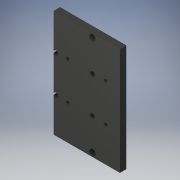
# Autodesk Inventor part: lidarCamMountv2
Saved by Autodesk Inventor 2017 (Build 210142000, 142)
## iProperties
Created: 2017-03-03
Part Number: lidarCamMountv2
Material: ABS Plastic
Document SubType Name: Modeling
Designer: Naga
Density: 1.06 g/cm^3
Appearance: Smooth - Black
Author: Naga
Autodesk Inventor part; units mm, degrees
ref_plane "YZ Plane" through (0, 0, 0) normal (1, 0, 0) x (0, 1, 0)
ref_plane "XZ Plane" through (0, 0, 0) normal (0, 1, 0) x (-1, 0, 0)
ref_plane "XY Plane" through (0, 0, 0) normal (0, 0, 1) x (1, 0, 0)
sketch "Sketch1" plane through (0, 0, 0) normal (0, 0, 1) x (1, 0, 0)
  line L0 (-33.3375, -53.975) -> (33.3375, -53.975)
  line L1 (33.3375, -53.975) -> (33.3375, 53.975)
  line L2 (33.3375, 53.975) -> (-33.3375, 53.975)
  line L3 (-33.3375, 53.975) -> (-33.3375, -53.975)
  line L4 (-33.3375, -53.975) -> (33.3375, 53.975) construction
  line L5 (33.3375, -53.975) -> (-33.3375, 53.975) construction
  point P0 (0, 0)
  dimension "d0" = 66.675
  dimension "d1" = 107.95
  constraints: 12 end point, 2 midpoint, 2 parallel, 1 horizontal, 1 perpendicular
  measures "d0" distance of L2.end L1.end
  measures "d1" distance of L1.end L0.end
extrude "Extrusion1" add sketch "Sketch1" along normal blind 6.35
sketch "Sketch3" plane through (0, 0, 6.35) normal (0, 0, 1) x (1, 0, 0)
  line L0 (-19.05, -19.05) -> (19.05, -19.05)
  line L1 (19.05, -19.05) -> (19.05, 19.05)
  line L2 (19.05, 19.05) -> (-19.05, 19.05)
  line L3 (-19.05, 19.05) -> (-19.05, -19.05)
  line L4 (-19.05, -19.05) -> (19.05, 19.05) construction
  line L5 (19.05, -19.05) -> (-19.05, 19.05) construction
  line L6 (0, 0) -> (-12.7, 0)
  line L7 (-31.115, -18.415) -> (5.715, -18.415)
  line L8 (5.715, -18.415) -> (5.715, 18.415)
  line L9 (5.715, 18.415) -> (-31.115, 18.415)
  line L10 (-31.115, 18.415) -> (-31.115, -18.415)
  line L11 (-31.115, -18.415) -> (5.715, 18.415) construction
  line L12 (5.715, -18.415) -> (-31.115, 18.415) construction
  circle A0 centre (19.05, 19.05) radius 1.5875
  circle A1 centre (19.05, -19.05) radius 1.5875
  circle A2 centre (-19.05, 19.05) radius 1.5875
  circle A3 centre (-19.05, -19.05) radius 1.5875
  circle A4 centre (5.715, 18.415) radius 1.5875
  circle A5 centre (5.715, -18.415) radius 1.5875
  circle A6 centre (-31.115, 18.415) radius 1.5875
  circle A7 centre (-31.115, -18.415) radius 1.5875
  line L13 (5.715, 18.415) -> (5.715, 50.165)
  circle A8 centre (5.715, 50.165) radius 3.175
  line L14 (5.715, -18.415) -> (5.715, -50.165)
  circle A9 centre (5.715, -50.165) radius 3.175
  dimension "d11" = 38.1
  dimension "d12" = 38.1
  dimension "d13" = 12.7
  dimension "d14" = 36.83
  dimension "d15" = 36.83
  dimension "d16" = 3.175
  dimension "d17" = 3.175
  dimension "d18" = 3.175
  dimension "d19" = 3.175
  dimension "d20" = 3.175
  dimension "d21" = 3.175
  dimension "d22" = 3.175
  dimension "d23" = 3.175
  dimension "d24" = 31.75
  dimension "d25" = 6.35
  dimension "d26" = 31.75
  dimension "d27" = 6.35
  constraints: 30 end point, 10 centre point, 10 coincident, 4 midpoint, 4 parallel, 4 perpendicular, 2 horizontal, 1 vertical
  measures "d11" distance of L2.end L1.end
  measures "d12" distance of L1.end L0.end
  measures "d13" distance of L6.start L6.end
  measures "d14" distance of L9.end L8.end
  measures "d15" distance of L8.end L7.end
  measures "d16" diameter of A0
  measures "d17" diameter of A1
  measures "d18" diameter of A2
  measures "d19" diameter of A3
  measures "d20" diameter of A4
  measures "d21" diameter of A5
  measures "d22" diameter of A6
  measures "d23" diameter of A7
  measures "d24" distance of L8.end L13.end
  measures "d25" diameter of A8
  measures "d26" distance of L14.start L14.end
  measures "d27" diameter of A9
extrude "Extrusion2" cut sketch "Sketch3" against normal blind 6.35 contours L3 L7 A3 L0 | L0 A3 L7 L3 | A8 | A9 | L7 A3 L3 | L3 A3 L7 | A5 L7 L14 L0 | L0 L14 A5 | L14 L8 A5 L0 | L0 A5 L14 | A5 L8 L7 | A7 L10 L7 | L7 L10 A7 | A2 L9 L3 | L3 L9 A2 | L9 A2 L2 L3 | L3 L2 A2 L9 | A1 L1 L0 | L0 L1 A1 | A4 L9 L8 | L8 L13 L2 A4 | A6 L9 L10 | L10 L9 A6 | A4 L2 L13 L9 | A4 L13 L2 | A0 L2 L1 | L1 L2 A0 | L13 A4 L2
sketch "Sketch4" plane through (0, 0, 6.35) normal (0, 0, 1) x (1, 0, 0)
  circle A0 centre (-31.115, 18.415) radius 1.5875 projected
  circle A1 centre (-31.115, -18.415) radius 1.5875 projected
  circle A2 centre (5.715, -18.415) radius 1.5875 projected
  circle A3 centre (5.715, 18.415) radius 1.5875 projected
  circle A4 centre (-31.115, 18.415) radius 2.3812
  circle A5 centre (-31.115, -18.415) radius 2.3813
  circle A6 centre (5.715, -18.415) radius 2.3812
  circle A7 centre (5.715, 18.415) radius 2.3813
  point P0 (0, 0)
  dimension "d30" = 4.7625
  dimension "d31" = 4.7625
  dimension "d32" = 4.7625
  dimension "d33" = 4.7625
  constraints: 4 centre point, 4 coincident
  measures "d30" diameter of A4
  measures "d31" diameter of A5
  measures "d32" diameter of A6
  measures "d33" diameter of A7
extrude "Extrusion3" cut sketch "Sketch4" against normal blind 3.175
sketch "Sketch5" plane through (0, 0, 0) normal (0, 0, -1) x (-1, 0, 0)
  circle A0 centre (19.05, 19.05) radius 1.5875 projected
  circle A1 centre (19.05, -19.05) radius 1.5875 projected
  circle A2 centre (-19.05, -19.05) radius 1.5875 projected
  circle A3 centre (-19.05, 19.05) radius 1.5875 projected
  line L0 (-16.3004, 19.05) -> (-17.6752, 16.6687)
  line L1 (-17.6752, 16.6687) -> (-20.4248, 16.6687)
  line L2 (-20.4248, 16.6687) -> (-21.7996, 19.05)
  line L3 (-21.7996, 19.05) -> (-20.4248, 21.4312)
  line L4 (-20.4248, 21.4312) -> (-17.6752, 21.4313)
  line L5 (-17.6752, 21.4313) -> (-16.3004, 19.05)
  line L6 (-33.3375, 53.975) -> (33.3375, 53.975) projected
  line L7 (-33.3375, -53.975) -> (-33.3375, 53.975) projected
  line L8 (-16.3004, -19.05) -> (-17.6752, -21.4313)
  line L9 (-17.6752, -21.4313) -> (-20.4248, -21.4313)
  line L10 (-20.4248, -21.4313) -> (-21.7996, -19.05)
  line L11 (-21.7996, -19.05) -> (-20.4248, -16.6688)
  line L12 (-20.4248, -16.6688) -> (-17.6752, -16.6687)
  line L13 (-17.6752, -16.6687) -> (-16.3004, -19.05)
  line L14 (21.7996, 19.05) -> (20.4248, 16.6687)
  line L15 (20.4248, 16.6687) -> (17.6752, 16.6687)
  line L16 (17.6752, 16.6687) -> (16.3004, 19.05)
  line L17 (16.3004, 19.05) -> (17.6752, 21.4312)
  line L18 (17.6752, 21.4312) -> (20.4248, 21.4312)
  line L19 (20.4248, 21.4312) -> (21.7996, 19.05)
  line L20 (21.7996, -19.05) -> (20.4248, -21.4313)
  line L21 (20.4248, -21.4313) -> (17.6752, -21.4313)
  line L22 (17.6752, -21.4313) -> (16.3004, -19.05)
  line L23 (16.3004, -19.05) -> (17.6752, -16.6688)
  line L24 (17.6752, -16.6688) -> (20.4248, -16.6688)
  line L25 (20.4248, -16.6688) -> (21.7996, -19.05)
  point P0 (0, 0)
  point P1 (-19.05, -19.05)
  point P2 (19.05, 19.05)
  point P3 (19.05, -19.05)
  dimension "d36" = 4.7625
  dimension "d39" = 38.1
  dimension "d42" = 38.1
  constraints: 48 end point, 1 coincident, 1 horizontal, 1 vertical, 52 other
  measures "d36" distance between parallel lines of L3 L0
  measures "d39" distance of point (-19.05, 19.05) point (-19.05, -19.05)
  measures "d42" distance of point (-19.05, 19.05) point (19.05, 19.05)
extrude "Extrusion4" cut sketch "Sketch5" against normal blind 1.5875
body "Solid1"
